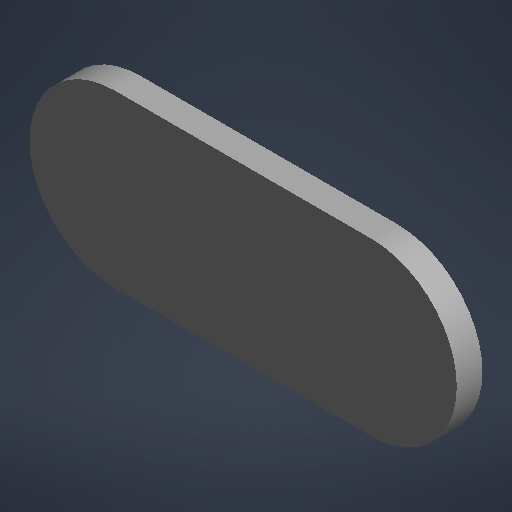
# Autodesk Inventor part: test_internal_holes_cad_model
Saved by Autodesk Inventor 2026 (Build 300175050, 175E)
## iProperties
Part Number: test_internal_holes_cad_model
Material: Generic
Document SubType Name: Modeling
Designer: Administrator
Appearance: Default
Author: Administrator
Autodesk Inventor part; units mm, degrees
ref_plane "YZ Plane" through (0, 0, 0) normal (1, 0, 0) x (0, 1, 0)
ref_plane "XZ Plane" through (0, 0, 0) normal (0, 1, 0) x (-1, 0, 0)
ref_plane "XY Plane" through (0, 0, 0) normal (0, 0, 1) x (1, 0, 0)
sketch "Sketch1" plane through (0, 0, 0) normal (0, 0, 1) x (1, 0, 0)
  arc A0 (2, 7) -> (2, 3) centre (2, 5) ccw
  line L0 (2, 3) -> (8, 3)
  arc A1 (8, 3) -> (8, 7) centre (8, 5) ccw
  line L1 (2, 7) -> (8, 7)
  constraints: 4 end point, 4 point on circle, 2 centre point
extrude "Extrusion1" add sketch "Sketch1" along normal blind 0.6
body "Solid1"
